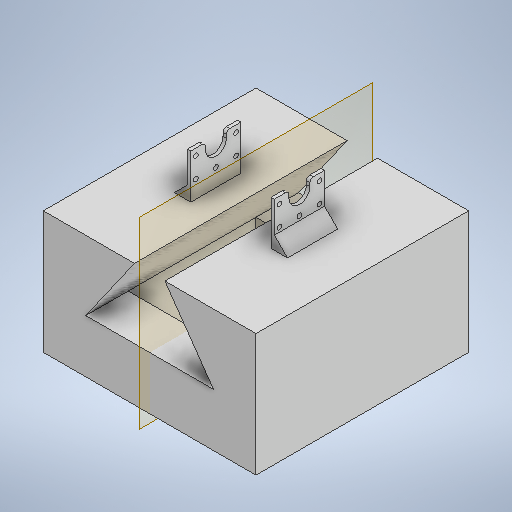
# Autodesk Inventor part: ADAPTER4BB
Saved by Autodesk Inventor 2027 (Build 310192060, 192F)
## iProperties
Created: 2026-07-14
Part Number: ADAPTER4BB
Material: Generic
Document SubType Name: Modeling
Designer: 13129
Density: 1 g/cm^3
Appearance: Default
Author: 13129
Autodesk Inventor part; units mm, degrees
ref_plane "XZ Plane" through (0, 0, 0) normal (0, 1, 0) x (-1, 0, 0)
ref_plane "XY Plane" through (0, 0, 0) normal (0, 0, 1) x (1, 0, 0)
sketch "Sketch1" plane through (0, 0, 0) normal (0, 1, 0) x (-1, 0, 0)
  line L0 (-38.25, 38.25) -> (38.25, 38.25)
  line L1 (38.25, 38.25) -> (38.25, -38.25)
  line L2 (38.25, -38.25) -> (-38.25, -38.25)
  line L3 (-38.25, -38.25) -> (-38.25, 38.25)
  line L4 (63.65, -63.65) -> (-63.65, -63.65)
  line L5 (-63.65, -63.65) -> (-63.65, 63.65)
  line L6 (-63.65, 63.65) -> (63.65, 63.65)
  line L7 (63.65, 63.65) -> (63.65, -63.65)
  point P0 (0, 0)
  point P1 (38.25, 0)
  point P2 (0, -38.25)
  point P3 (63.65, 0)
  point P4 (0, -63.65)
  dimension "d0" = 76.5
  dimension "d1" = 76.5
  dimension "d2" = 25.4
  dimension "d3" = 25.4
  constraints: 16 end point, 4 midpoint, 4 parallel, 2 horizontal, 2 horizontal alignment, 2 perpendicular, 2 vertical alignment
  measures "d0" distance of L1.end L2.end
  measures "d1" distance of L0.end L1.end
  measures "d2" distance between parallel lines of L7 L1
  measures "d3" distance between parallel lines of L4 L2
extrude "Extrusion1" add sketch "Sketch1" along normal blind 31.75
sketch "Sketch2" plane through (-63.65, 0, 63.65) normal (0, 0, 1) x (1, 0, 0)
  line L0 (127.3, 0) -> (127.3, 31.75) construction
  line L1 (0, 31.75) -> (127.3, 31.75) construction
  line L2 (101.9, 0) -> (101.9, 31.75) construction
  line L3 (101.9, 31.75) -> (72.7623, 73.3629)
  line L4 (101.9, 31.75) -> (152.7, 31.75) construction
  line L5 (63.65, 0) -> (63.65, 31.75)
  line L6 (72.7623, 73.3629) -> (127.3, 73.3629)
  line L7 (127.3, 73.3629) -> (127.3, 31.75)
  line L8 (25.4, 31.75) -> (54.5377, 73.3629)
  line L9 (25.4, 31.75) -> (-25.4, 31.75) construction
  line L10 (54.5377, 73.3629) -> (0, 73.3629)
  line L11 (0, 73.3629) -> (0, 31.75)
  line L12 (0, 31.75) -> (127.3, 31.75)
  dimension "d6" = 125
  dimension "d7" = 50.8
  constraints: 20 end point, 4 symmetric about line, 2 perpendicular, 1 collinear, 1 equal length, 1 horizontal, 1 midpoint, 1 point on line
  measures "d6" angle of L4 L3
  measures "d7" distance of L2.end L3.end
extrude "Extrusion2" add sketch "Sketch2" against normal up to surface (127.3 mm away)
sketch "Sketch3" plane through (9.1123, 73.3629, 63.65) normal (0, 1, 0) x (1, 0, 0)
  line L0 (-33.1123, 48.65) -> (-33.1123, 78.65)
  line L1 (-33.1123, 78.65) -> (-35.1123, 78.65)
  line L2 (-35.1123, 78.65) -> (-35.1123, 48.65)
  line L3 (-35.1123, 48.65) -> (-33.1123, 48.65)
  line L4 (16.8877, 48.65) -> (16.8877, 78.65)
  line L5 (16.8877, 78.65) -> (14.8877, 78.65)
  line L6 (14.8877, 78.65) -> (14.8877, 48.65)
  line L7 (14.8877, 48.65) -> (16.8877, 48.65)
  line L8 (-18.2246, 0) -> (-18.2246, 127.3) construction
  line L9 (-33.1123, 63.65) -> (14.8877, 63.65) construction
  point P0 (-9.1123, 63.65)
  point P1 (-18.2246, 63.65)
  point P2 (-9.1123, 63.65)
  dimension "d10" = 30
  dimension "d11" = 2
  dimension "d12" = 30
  dimension "d13" = 2
  dimension "d14" = 48
  constraints: 18 end point, 4 midpoint, 4 perpendicular, 2 horizontal alignment, 2 parallel, 2 vertical, 1 coincident, 1 horizontal
  measures "d10" distance of L1.end L2.end
  measures "d11" distance of L0.end L1.end
  measures "d12" distance of L5.end L6.end
  measures "d13" distance of L4.end L5.end
  measures "d14" distance of L5.end L0.end
extrude "Extrusion3" add sketch "Sketch3" along normal blind 2
sketch "Sketch4" plane through (-26, 73.3629, 15) normal (-1, 0, 0) x (0, 0, 1)
  line L0 (0, 0) -> (-30, 0) construction
  line L1 (-30, 2) -> (0, 2) construction
  line L2 (0, 2) -> (-30, 2) construction
  line L3 (0, 2) -> (0, 26.5)
  line L4 (-30, 0) -> (0, 0) construction
  line L5 (0, 0) -> (-30, 0)
  line L6 (-30, 0) -> (-30, 2)
  line L7 (0, 0) -> (0, 2)
  line L8 (-30, 2) -> (0, 2)
  line L9 (-30, 2) -> (-30, 26.5)
  arc A0 (-21.25, 22.5) -> (-8.75, 22.5) centre (-15, 22.5) ccw
  line L10 (-21.25, 22.5) -> (-21.25, 24.5)
  line L11 (-8.75, 22.5) -> (-8.75, 24.5)
  line L12 (-30, 26.5) -> (-23.25, 26.5)
  line L13 (0, 26.5) -> (-6.75, 26.5)
  arc A1 (-21.25, 24.5) -> (-23.25, 26.5) centre (-23.25, 24.5) ccw
  arc A2 (-6.75, 26.5) -> (-8.75, 24.5) centre (-6.75, 24.5) ccw
  circle A3 centre (-3, 22.5) radius 1.4
  circle A4 centre (-3, 10.5) radius 1.4
  circle A5 centre (-15, 10.5) radius 1.4
  circle A6 centre (-27, 10.5) radius 1.4
  circle A7 centre (-27, 22.5) radius 1.4
  line L14 (-27, 10.5) -> (-15, 10.5) construction
  line L15 (-15, 10.5) -> (-3, 10.5) construction
  point P0 (-15, -73.3629)
  point P1 (-15, 2)
  point P2 (-15, 16.25)
  dimension "d17" = 26.5
  dimension "d18" = 12.5
  dimension "d19" = 22.5
  dimension "d20" = 2
  dimension "d21" = 2.8
  dimension "d22" = 12
  dimension "d23" = 24
  constraints: 24 end point, 8 centre point, 7 point on circle, 6 tangent, 5 equal radius, 5 horizontal alignment, 4 perpendicular, 4 vertical, 4 vertical alignment, 3 collinear, 2 horizontal, 1 midpoint
  measures "d17" distance from line of L3.end L0
  measures "d18" diameter of A0
  measures "d19" distance from line of L0 A0.centre
  measures "d20" radius of A1
  measures "d21" diameter of A3
  measures "d22" distance of L14.start A7.centre
  measures "d23" distance of L15.end L14.start
extrude "Extrusion4" add sketch "Sketch4" against normal blind 2 contours L8 L9 L12 A1 L10 A0 L11 A2 L13 L3
sketch "Sketch5" plane through (-24, 73.3629, -15) normal (0, 0, -1) x (-1, 0, 0)
  line L0 (2, 0) -> (0, 0) construction
  line L1 (1, 8.89) -> (9.89, 0)
  line L2 (-14.8877, 0) -> (39.65, 0) construction
  line L3 (1, 8.89) -> (13.5724, 8.89) construction
  line L4 (1, 8.89) -> (-7.89, 0)
  line L5 (1, 8.89) -> (13.5724, 8.89) construction
  line L6 (1, 8.89) -> (1, 0)
  line L7 (1, 0) -> (9.89, 0)
  point P0 (-24, -73.3629)
  dimension "d26" = 45
  dimension "d27" = 135
  dimension "d28" = 8.89
  constraints: 12 end point, 2 equal length, 2 horizontal, 2 midpoint, 2 point on line, 1 vertical, 1 vertical alignment
  measures "d26" angle of L1 L3
  measures "d27" angle of L4 L5
  measures "d28" distance of L6.end L1.start
extrude "Extrusion5" add sketch "Sketch5" against normal up to surface (30 mm away)
mirror "Mirror1" about plane through (0, 0, 0) normal (1, 0, 0) of "Extrusion4", "Extrusion5"
body "Solid1"
